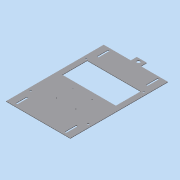
# Autodesk Inventor part: Innengehäuse
Saved by Autodesk Inventor 2015 SP1 (Build 190203100, 203)
## iProperties
Created: 2015-04-13
Part Number: Innengehäuse
Material: Generisch
Document SubType Name: Modeling
Designer: ElMatinho
Density: 1 g/cm^3
Appearance: Vorgabe
Author: ElMatinho
Autodesk Inventor part; units mm, degrees
ref_plane "YZ Plane" through (0, 0, 0) normal (1, 0, 0) x (0, 1, 0)
ref_plane "XZ Plane" through (0, 0, 0) normal (0, 1, 0) x (-1, 0, 0)
ref_plane "XY Plane" through (0, 0, 0) normal (0, 0, 1) x (1, 0, 0)
sketch "Skizze1" plane through (0, 0, 0) normal (0, 0, 1) x (1, 0, 0)
  line L0 (-135.1, 0) -> (135.1, 0) projected
  line L1 (0, -215.3) -> (0, 220.8) projected
  line L2 (15, 140.5) -> (15, 158.5)
  line L3 (15, 158.5) -> (-15, 158.5)
  line L4 (-15, 158.5) -> (-15, 140.5)
  line L5 (-15, 140.5) -> (-96.5, 140.5)
  line L6 (-96.5, 140.5) -> (-96.5, -153)
  line L7 (-96.5, -153) -> (96.5, -153)
  line L8 (96.5, -153) -> (96.5, 140.5)
  line L9 (96.5, 140.5) -> (15, 140.5)
  circle A0 centre (86.5, 78) radius 2.5
  circle A1 centre (-86.5, 78) radius 2.5
  circle A2 centre (-86.5, -89) radius 2.5
  circle A3 centre (86.5, -89) radius 2.5
  arc A4 (-71.5, 132) -> (-76.5, 132) centre (-74, 132) ccw
  line L10 (-76.5, 132) -> (-76.5, 101.5)
  arc A5 (-76.5, 101.5) -> (-71.5, 101.5) centre (-74, 101.5) ccw
  line L11 (-71.5, 101.5) -> (-71.5, 132)
  arc A6 (76.5, 132) -> (71.5, 132) centre (74, 132) ccw
  line L12 (76.5, 132) -> (76.5, 101.5)
  arc A7 (71.5, 101.5) -> (76.5, 101.5) centre (74, 101.5) ccw
  line L13 (71.5, 101.5) -> (71.5, 132)
  line L14 (-80.5, 75) -> (80.5, 75)
  line L15 (80.5, 75) -> (80.5, 0)
  line L16 (80.5, 0) -> (-80.5, 0)
  line L17 (-80.5, 0) -> (-80.5, 75)
  circle A8 centre (29, -20) radius 1.25
  circle A9 centre (-29, -20) radius 1.25
  circle A10 centre (-29, -69) radius 1.25
  circle A11 centre (29, -69) radius 1.25
  arc A12 (-71.5, -112.5) -> (-76.5, -112.5) centre (-74, -112.5) ccw
  line L18 (-76.5, -112.5) -> (-76.5, -143)
  arc A13 (-76.5, -143) -> (-71.5, -143) centre (-74, -143) ccw
  line L19 (-71.5, -143) -> (-71.5, -112.5)
  arc A14 (76.5, -112.5) -> (71.5, -112.5) centre (74, -112.5) ccw
  line L20 (76.5, -112.5) -> (76.5, -143)
  arc A15 (71.5, -143) -> (76.5, -143) centre (74, -143) ccw
  line L21 (71.5, -143) -> (71.5, -112.5)
  circle A16 centre (0, 148.5) radius 5
  point P0 (0, 0)
  dimension "d0" = 30
  dimension "d1" = 193
  dimension "d2" = 293.5
  dimension "d3" = 65.5
  dimension "d4" = 75
  dimension "d5" = 16
  dimension "d6" = 16
  dimension "d7" = 65.5
  dimension "d9" = 148
  dimension "d10" = 5
  dimension "d11" = 2.5
  dimension "d12" = 2.5
  dimension "d13" = 30.5
  dimension "d14" = 8.5
  dimension "d15" = 5
  dimension "d16" = 30.5
  dimension "d17" = 2.5
  dimension "d18" = 2.5
  dimension "d19" = 143
  dimension "d20" = 6
  dimension "d21" = 3
  dimension "d22" = 6
  dimension "d23" = 3
  dimension "d24" = 75
  dimension "d25" = 167
  dimension "d26" = 10
  dimension "d27" = 167
  dimension "d28" = 10
  dimension "d29" = 20
  dimension "d30" = 8.5
  dimension "d31" = 81.5
  dimension "d32" = 58
  dimension "d33" = 49
  dimension "d34" = 58
  dimension "d35" = 49
  dimension "d36" = 67.5
  dimension "d37" = 67.5
  dimension "d38" = 67.5
  dimension "d39" = 20
  dimension "d40" = 84
  dimension "d41" = 5
  dimension "d42" = 5
  dimension "d43" = 2.5
  dimension "d44" = 2.5
  dimension "d45" = 2.5
  dimension "d46" = 2.5
  dimension "d47" = 5
  dimension "d48" = 5
  dimension "d49" = 2.5
  dimension "d50" = 2.5
  dimension "d51" = 2.5
  dimension "d52" = 2.5
  dimension "d53" = 30.5
  dimension "d54" = 30.5
  dimension "d55" = 5
  dimension "d56" = 5
  dimension "d57" = 10
  dimension "d58" = 10
  dimension "d59" = 22.5
  dimension "d60" = 22.5
  dimension "d61" = 22.5
  dimension "d62" = 22.5
  dimension "d63" = 143
  dimension "d65" = 18
  constraints: 40 end point, 17 centre point, 16 point on circle, 1 midpoint, 1 point on line, 1 other
  measures "d0" distance of L2.end L3.end
  measures "d1" distance between parallel lines of L8 L6
  measures "d2" distance of L7.end L8.end
  measures "d3" distance between parallel lines of L14 L9
  measures "d4" distance of L14.end L15.end
  measures "d5" distance between parallel lines of L8 L15
  measures "d6" distance between parallel lines of L6 L17
  measures "d7" distance between parallel lines of L5 L14
  measures "d9" distance of A6.centre A4.centre
  measures "d10" distance between parallel lines of L11 L10
  measures "d11" radius of A5
  measures "d12" radius of A4
  measures "d13" distance of A4.centre A5.centre
  measures "d14" distance from line of L5 A4.centre
  measures "d15" distance between parallel lines of L12 L13
  measures "d16" distance of A6.centre A7.centre
  measures "d17" radius of A7
  measures "d18" radius of A6
  measures "d19" distance between parallel lines of L11 L13
  measures "d20" distance from line of L17 A1.centre
  measures "d21" distance from line of L14 A1.centre
  measures "d22" distance from line of L15 A0.centre
  measures "d23" distance from line of L14 A0.centre
  measures "d24" distance between parallel lines of L16 L14
  measures "d25" distance of A2.centre A1.centre
  measures "d26" distance from line of L6 A2.centre
  measures "d27" distance of A3.centre A0.centre
  measures "d28" distance from line of L8 A3.centre
  measures "d29" distance between parallel lines of L6 L10
  measures "d30" distance from line of L9 A6.centre
  measures "d31" distance between parallel lines of L4 L6
  measures "d32" distance of A8.centre A9.centre
  measures "d33" distance of A10.centre A9.centre
  measures "d34" distance of A11.centre A10.centre
  measures "d35" distance of A8.centre A11.centre
  measures "d36" distance from line of L8 A8.centre
  measures "d37" distance from line of L8 A11.centre
  measures "d38" distance from line of L6 A9.centre
  measures "d39" distance from line of L16 A9.centre
  measures "d40" distance from line of L7 A10.centre
  measures "d41" diameter of A1
  measures "d42" diameter of A0
  measures "d43" diameter of A9
  measures "d44" diameter of A8
  measures "d45" diameter of A10
  measures "d46" diameter of A11
  measures "d47" diameter of A2
  measures "d48" diameter of A3
  measures "d49" radius of A12
  measures "d50" radius of A13
  measures "d51" radius of A14
  measures "d52" radius of A15
  measures "d53" distance of A13.centre A12.centre
  measures "d54" distance of A14.centre A15.centre
  measures "d55" distance between parallel lines of L18 L19
  measures "d56" distance between parallel lines of L20 L21
  measures "d57" distance from line of L7 A13.centre
  measures "d58" distance from line of L7 A15.centre
  measures "d59" distance from line of L6 A13.centre
  measures "d60" distance from line of L6 A12.centre
  measures "d61" distance from line of L8 A14.centre
  measures "d62" distance from line of L8 A15.centre
  measures "d63" distance between parallel lines of L21 L19
  measures "d65" distance between parallel lines of L3 L9
extrude "Extrusion1" add sketch "Skizze1" along normal blind 1.5 contours L6 L5 L4 L3 L1 A16 L14 L17 L0 | L0 L1 L7 L6 | L0 L8 L7 L1 | L15 L14 L1 A16 L3 L2 L9 L8 L0
